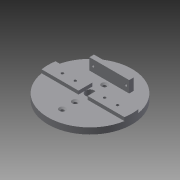
# Autodesk Inventor part: Master Tablet and IR Mount
Saved by Autodesk Inventor 2014 SP2 (Build 180246200, 246)
## iProperties
Created: 2015-08-19
Part Number: Master Tablet and IR Mount
Material: Generic
Document SubType Name: Modeling
Designer: Devon
Density: 1 g/cm^3
Appearance: Default
Author: Devon
Autodesk Inventor part; units mm, degrees
ref_plane "YZ Plane" through (0, 0, 0) normal (1, 0, 0) x (0, 1, 0)
ref_plane "XZ Plane" through (0, 0, 0) normal (0, 1, 0) x (-1, 0, 0)
ref_plane "XY Plane" through (0, 0, 0) normal (0, 0, 1) x (1, 0, 0)
sketch "Sketch1" plane through (0, 0, 0) normal (0, 1, 0) x (-1, 0, 0)
  circle A0 centre (0, 0) radius 46.99
  line L0 (0, 0) -> (16.383, 0)
  line L1 (16.383, 0) -> (30.861, 0)
  line L2 (0, 0) -> (0, -16.383)
  line L3 (0, -16.383) -> (0, -30.861)
  line L4 (0, 0) -> (0, 16.383)
  line L5 (0, 16.383) -> (0, 30.861)
  line L6 (0, 0) -> (-16.383, 0)
  line L7 (-16.383, 0) -> (-30.861, 0)
  circle A1 centre (0, 30.861) radius 1.905
  circle A2 centre (30.861, 0) radius 1.4732
  circle A3 centre (0, -30.861) radius 1.905
  circle A4 centre (-30.861, 0) radius 1.4732
  circle A5 centre (-16.383, 0) radius 1.4732
  circle A6 centre (0, 16.383) radius 1.905
  circle A7 centre (16.383, 0) radius 1.4732
  circle A8 centre (0, -16.383) radius 1.905
  dimension "d0" = 93.98
  dimension "d1" = 16.383
  dimension "d2" = 14.478
  dimension "d3" = 16.383
  dimension "d4" = 14.478
  dimension "d5" = 16.383
  dimension "d6" = 14.478
  dimension "d7" = 16.383
  dimension "d8" = 14.478
  dimension "d9" = 3.81
  dimension "d10" = 2.9464
  dimension "d11" = 3.81
  dimension "d12" = 2.9464
  dimension "d13" = 2.9464
  dimension "d14" = 3.81
  dimension "d15" = 2.9464
  dimension "d16" = 3.81
  constraints: 16 end point, 9 centre point, 9 coincident, 5 collinear, 2 perpendicular, 1 horizontal
  measures "d0" diameter of A0
  measures "d1" distance of L0.start L0.end
  measures "d2" distance of L0.end L1.end
  measures "d3" distance of L0.start L2.end
  measures "d4" distance of L2.end L3.end
  measures "d5" distance of L0.start L4.end
  measures "d6" distance of L4.end L5.end
  measures "d7" distance of L0.start L6.end
  measures "d8" distance of L6.end L7.end
  measures "d9" diameter of A1
  measures "d10" diameter of A2
  measures "d11" diameter of A3
  measures "d12" diameter of A4
  measures "d13" diameter of A5
  measures "d14" diameter of A6
  measures "d15" diameter of A7
  measures "d16" diameter of A8
extrude "Extrusion1" add sketch "Sketch1" along normal blind 6.858
sketch "Sketch2" plane through (0, 6.858, 0) normal (0, 1, 0) x (1, 0, 0)
  circle A0 centre (0, 0) radius 46.99 projected
hole "Hole1" at (0, 6.858, 0) direction (0, -1, 0) diameter 10.16 depth 25.4 tip angle 118
sketch "Sketch3" plane through (0, 6.858, 0) normal (0, 1, 0) x (1, 0, 0)
  circle A0 centre (-16.383, 0) radius 1.4732 projected
  circle A1 centre (16.383, 0) radius 1.4732 projected
  circle A2 centre (30.861, 0) radius 1.4732 projected
  circle A3 centre (-30.861, 0) radius 1.4732 projected
  circle A4 centre (0, 0) radius 46.99 projected
  line L0 (0, 0) -> (0, 7.8105)
  line L1 (0, 0) -> (0, -7.8105)
  line L2 (0, -7.8105) -> (46.3363, -7.8105)
  line L3 (0, 7.8105) -> (46.3363, 7.8105)
  line L4 (0, 7.8105) -> (-46.3363, 7.8105)
  line L5 (0, -7.8105) -> (-46.3363, -7.8105)
  line L6 (-5.08, -7.8105) -> (-5.08, 7.8105)
  line L7 (5.08, -7.8105) -> (5.08, 7.8105)
  dimension "d26" = 7.8105
  dimension "d27" = 7.8105
  constraints: 16 end point, 4 equal length, 4 point on circle, 4 point on line, 3 perpendicular, 1 vertical
  measures "d26" distance of L0.start L0.end
  measures "d27" distance of L0.start L1.end
extrude "Extrusion2" add sketch "Sketch3" along normal blind 3.81 contours A4 L2 L7 L3 | L4 L6 L5 A4
chamfer "Chamfer1" distance 1.5875 angle 45 1 edges at (1.905, 6.858, 30.861)
chamfer "Chamfer2" distance 1.5875 angle 45 3 edges at (1.905, 6.858, 16.383) (1.905, 6.858, -16.383) (1.905, 6.858, -30.861)
sketch "Sketch4" plane through (0, 6.858, 0) normal (0, 1, 0) x (1, 0, 0)
  line L0 (0, 21.59) -> (22.225, 21.59)
  line L1 (0, 21.59) -> (-22.225, 21.59)
  line L2 (-22.225, 21.59) -> (-22.225, 26.67)
  line L3 (-22.225, 26.67) -> (22.225, 26.67)
  line L4 (22.225, 26.67) -> (22.225, 21.59)
  dimension "d37" = 22.225
  dimension "d38" = 22.225
  dimension "d39" = 5.08
  constraints: 10 end point, 2 equal length, 2 perpendicular
  measures "d37" distance of L0.start L0.end
  measures "d38" distance of L0.start L1.end
  measures "d39" distance of L1.end L2.end
extrude "Extrusion3" add sketch "Sketch4" along normal blind 12.954
sketch "Sketch5" plane through (22.225, 6.858, -26.67) normal (0, 0, -1) x (-1, 0, 0)
  line L0 (44.45, 0) -> (44.45, 12.954) projected
  line L1 (0, 0) -> (0, 12.954) projected
  line L2 (0, 6.477) -> (44.45, 6.477)
  line L3 (44.45, 6.477) -> (40.64, 6.477)
  line L4 (0, 6.477) -> (3.81, 6.477)
  circle A0 centre (3.81, 6.477) radius 1.524
  circle A1 centre (40.64, 6.477) radius 1.524
  point P0 (22.225, -6.858)
  dimension "d42" = 3.81
  dimension "d43" = 3.81
  dimension "d44" = 3.048
  dimension "d45" = 3.048
  constraints: 6 end point, 2 centre point, 2 coincident, 2 midpoint, 2 point on line
  measures "d42" distance of L2.end L3.end
  measures "d43" distance of L2.start L4.end
  measures "d44" diameter of A0
  measures "d45" diameter of A1
hole "Hole2" at (18.415, 13.335, -26.67) at (-18.415, 13.335, -26.67) direction (0, 0, 1) diameter 3.048 depth 25.4 tip angle 118
body "Solid1"
